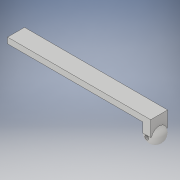
# Autodesk Inventor part: Maccaronistössel
Saved by Autodesk Inventor 2019 (Build 230136000, 136)
## iProperties
Created: 2022-03-16
Part Number: Maccaronistössel
Material: Generic
Document SubType Name: Modeling
Designer: Lukas
Density: 1 g/cm^3
Appearance: Default
Author: Lukas
Autodesk Inventor part; units mm, degrees
ref_plane "YZ Plane" through (0, 0, 0) normal (1, 0, 0) x (0, 1, 0)
ref_plane "XZ Plane" through (0, 0, 0) normal (0, 1, 0) x (-1, 0, 0)
ref_plane "XY Plane" through (0, 0, 0) normal (0, 0, 1) x (1, 0, 0)
sketch "Sketch1" plane through (0, 0, 0) normal (0, 0, 1) x (1, 0, 0)
  circle A0 centre (0, 0) radius 4.5
  line L0 (-4.5, 0) -> (4.5, 0)
  line L1 (-6.3, 0) -> (6.3, 0) projected
  dimension "d0" = 9
  constraints: 2 end point, 2 point on circle, 1 centre point, 1 coincident, 1 horizontal, 1 midpoint
  measures "d0" diameter of A0
revolve "Revolution1" add sketch "Sketch1" angle 360 about axis through (-10, 0, 0) along (1, 0, 0) picked at (0.8521, 1.2345) contours L0 A0
sketch "Sketch4" plane through (0, 0, 0) normal (0, 0, 1) x (1, 0, 0)
  circle A0 centre (0, 0) radius 1
  dimension "d15" = 2
  constraints: 1 centre point, 1 coincident
  measures "d15" diameter of A0
extrude "Extrusion4" cut sketch "Sketch4" along normal through all both and the other way through all
sketch "Sketch5" plane through (0, 0, 0) normal (1, 0, 0) x (0, 1, 0)
  line L0 (1, -4.3875) -> (1, 4.3875) projected
  line L1 (1, -4.3875) -> (9, -4.3875)
  line L2 (9, -4.3875) -> (9, 4.3875)
  line L3 (9, 4.3875) -> (1, 4.3875)
  line L4 (1, 4.3875) -> (1, -4.3875)
  point P0 (0, 0)
  point P1 (9, 0)
  dimension "d19" = 8
  constraints: 8 end point, 2 parallel, 1 horizontal, 1 horizontal alignment, 1 midpoint, 1 perpendicular
  measures "d19" distance of L2.end L3.end
extrude "Extrusion5" add sketch "Sketch5" along normal mid plane 4
sketch "Sketch6" plane through (-2, 0, 0) normal (-1, 0, 0) x (0, 0, 1)
  line L0 (4.3875, 9) -> (-4.3875, 9) projected
  line L1 (4.3875, 1) -> (4.3875, 9) projected
  line L2 (-4.3875, 9) -> (4.3875, 9)
  line L3 (4.3875, 9) -> (4.3875, 6)
  line L4 (4.3875, 6) -> (-4.3875, 6)
  line L5 (-4.3875, 6) -> (-4.3875, 9)
  point P0 (0, 0)
  dimension "d22" = 3
  constraints: 8 end point, 2 parallel, 1 horizontal, 1 perpendicular, 1 point on line
  measures "d22" distance between parallel lines of L2 L4
extrude "Extrusion6" add sketch "Sketch6" along normal blind 70
body "Solid2"
